Autodesk Inventor part; units mm, degrees
(part 7 of 7)
sketch "Esboço14" plane through (-80, -75, 4) normal (0, -1, 0) x (1, 0, 0)
  line L0 (170, 0) -> (160, 0) projected
  line L1 (160, 0) -> (160, -46)
  line L2 (160, -132) -> (160, 0) projected
  line L3 (160, 0) -> (206, 0) construction
  line L4 (160, -46) -> (0, -46)
  line L5 (0, 0) -> (0, -132) projected
  line L6 (160, -4) -> (160, 0) projected
  line L7 (160, 0) -> (160, -84)
  line L8 (160, 0) -> (244, 0) construction
  line L9 (160, -84) -> (0, -84)
  line L10 (160, -46) -> (160, -65)
  line L11 (160, -46) -> (179, -46) construction
  line L12 (160, -65) -> (125.67, -65)
  line L13 (125.67, -65) -> (103.67, -65)
  line L14 (103.67, -65) -> (69.34, -65)
  line L15 (69.34, -65) -> (34.34, -65)
  line L16 (69.34, -65) -> (104.34, -65) construction
  line L17 (34.34, -65) -> (0.01, -65)
  line L18 (124.67, -71.5) -> (104.67, -71.5)
  line L19 (104.67, -71.5) -> (104.67, -58.5)
  line L20 (104.67, -58.5) -> (124.67, -58.5)
  line L21 (124.67, -58.5) -> (124.67, -71.5)
  line L22 (124.67, -71.5) -> (104.67, -58.5) construction
  line L23 (104.67, -71.5) -> (124.67, -58.5) construction
  line L24 (62.24, -71.4) -> (41.44, -71.4)
  line L25 (41.44, -71.4) -> (41.44, -58.6)
  line L26 (41.44, -58.6) -> (62.24, -58.6)
  line L27 (62.24, -58.6) -> (62.24, -71.4)
  line L28 (62.24, -71.4) -> (41.44, -58.6) construction
  line L29 (41.44, -71.4) -> (62.24, -58.6) construction
  line L30 (160, -132) -> (160, -129)
  line L31 (160, -132) -> (163, -132) construction
  line L32 (160, -129) -> (0, -129)
  line L33 (160, -84) -> (160, -109.5)
  line L34 (160, -84) -> (185.5, -84) construction
  line L35 (160, -109.5) -> (150, -109.5)
  line L36 (150, -109.5) -> (85, -109.5)
  line L37 (85, -109.5) -> (65, -109.5)
  line L38 (65, -109.5) -> (53, -109.5)
  line L39 (117.5, -109.5) -> (117.5, -104.5)
  line L40 (140, -106.5) -> (95, -106.5)
  line L41 (95, -106.5) -> (95, -102.5)
  line L42 (95, -102.5) -> (140, -102.5)
  line L43 (140, -102.5) -> (140, -106.5)
  line L44 (140, -106.5) -> (95, -102.5) construction
  line L45 (95, -106.5) -> (140, -102.5) construction
  circle A0 centre (59, -109.5) radius 3.5
  point P0 (80, -4)
  point P1 (114.67, -65)
  point P2 (51.84, -65)
  dimension "d150" = 46
  dimension "d151" = 90
  dimension "d152" = 84
  dimension "d153" = 90
  dimension "d154" = 19
  dimension "d155" = 90
  dimension "d156" = 34.33
  dimension "d157" = 22
  dimension "d158" = 34.33
  dimension "d159" = 35
  dimension "d160" = 180
  dimension "d161" = 34.33
  dimension "d162" = 180
  dimension "d163" = 20
  dimension "d164" = 13
  dimension "d165" = 20.8
  dimension "d166" = 12.8
  dimension "d167" = 3
  dimension "d168" = 90
  dimension "d169" = 25.5
  dimension "d170" = 90
  dimension "d171" = 10
  dimension "d172" = 65
  dimension "d173" = 20
  dimension "d174" = 12
  dimension "d175" = 5
  dimension "d176" = 45
  dimension "d177" = 4
  dimension "d178" = 7
  constraints: 84 end point, 12 horizontal, 10 midpoint, 8 perpendicular, 6 equal length, 6 parallel, 6 point on line, 5 collinear, 1 centre point, 1 vertical
  measures "d150" distance of L0.end L1.end
  measures "d151" angle of L1 L3
  measures "d152" distance of L0.end L7.end
  measures "d153" angle of L7 L8
  measures "d154" distance of L1.end L10.end
  measures "d155" angle of L10 L11
  measures "d156" distance of L10.end L12.end
  measures "d157" distance of L12.end L13.end
  measures "d158" distance of L13.end L14.end
  measures "d159" distance of L14.end L15.end
  measures "d160" angle of L15 L16
  measures "d161" distance of L15.end L17.end
  measures "d162" angle of L17 L15
  measures "d163" distance of L19.end L20.end
  measures "d164" distance of L18.end L19.end
  measures "d165" distance of L25.end L26.end
  measures "d166" distance of L24.end L25.end
  measures "d167" distance of L2.start L30.end
  measures "d168" angle of L31 L30
  measures "d169" distance of L7.end L33.end
  measures "d170" angle of L33 L34
  measures "d171" distance of L33.end L35.end
  measures "d172" distance of L35.end L36.end
  measures "d173" distance of L36.end L37.end
  measures "d174" distance of L37.end L38.end
  measures "d175" distance of L39.start L39.end
  measures "d176" distance of L41.end L42.end
  measures "d177" distance of L40.end L41.end
  measures "d178" diameter of A0
extrude "Extrusão14" cut sketch "Esboço14" against normal blind 5 contours L21 L18 L19 L13 | L13 L19 L20 L21 | L27 L24 L25 L15 | L15 L25 L26 L27 | A0 L38 | L38 A0 | L40 L41 L42 L43
sketch "Esboço15" plane through (-80, -75, 4) normal (0, -1, 0) x (1, 0, 0)
  line L0 (170, 0) -> (160, 0)
  line L1 (160, 0) -> (160, -46)
  line L2 (160, -132) -> (160, 0)
  line L3 (160, 0) -> (206, 0) construction
  line L4 (160, -46) -> (0, -46)
  line L5 (0, 0) -> (0, -132)
  line L6 (160, -4) -> (160, 0)
  line L7 (160, 0) -> (160, -84)
  line L8 (160, 0) -> (244, 0) construction
  line L9 (160, -84) -> (0, -84)
  line L10 (160, -46) -> (160, -65)
  line L11 (160, -46) -> (179, -46) construction
  line L12 (160, -65) -> (125.67, -65)
  line L13 (125.67, -65) -> (103.67, -65)
  line L14 (103.67, -65) -> (69.34, -65)
  line L15 (69.34, -65) -> (34.34, -65)
  line L16 (69.34, -65) -> (104.34, -65) construction
  line L17 (34.34, -65) -> (0.01, -65)
  line L18 (124.67, -71.5) -> (104.67, -71.5)
  line L19 (104.67, -71.5) -> (104.67, -58.5)
  line L20 (104.67, -58.5) -> (124.67, -58.5)
  line L21 (124.67, -58.5) -> (124.67, -71.5)
  line L22 (124.67, -71.5) -> (104.67, -58.5) construction
  line L23 (104.67, -71.5) -> (124.67, -58.5) construction
  line L24 (62.24, -71.4) -> (41.44, -71.4)
  line L25 (41.44, -71.4) -> (41.44, -58.6)
  line L26 (41.44, -58.6) -> (62.24, -58.6)
  line L27 (62.24, -58.6) -> (62.24, -71.4)
  line L28 (62.24, -71.4) -> (41.44, -58.6) construction
  line L29 (41.44, -71.4) -> (62.24, -58.6) construction
  line L30 (160, -132) -> (160, -129)
  line L31 (160, -132) -> (163, -132) construction
  line L32 (160, -129) -> (0, -129)
  line L33 (160, -84) -> (160, -109.5)
  line L34 (160, -84) -> (185.5, -84) construction
  line L35 (160, -109.5) -> (150, -109.5)
  line L36 (150, -109.5) -> (85, -109.5)
  line L37 (85, -109.5) -> (65, -109.5)
  line L38 (65, -109.5) -> (53, -109.5)
  line L39 (117.5, -109.5) -> (117.5, -104.5)
  line L40 (140, -106.5) -> (95, -106.5)
  line L41 (95, -106.5) -> (95, -102.5)
  line L42 (95, -102.5) -> (140, -102.5)
  line L43 (140, -102.5) -> (140, -106.5)
  line L44 (140, -106.5) -> (95, -102.5) construction
  line L45 (95, -106.5) -> (140, -102.5) construction
  circle A0 centre (59, -109.5) radius 3.5
  line L46 (65.59, -65.5) -> (38.09, -65.5)
  line L47 (38.09, -65.5) -> (38.09, -64.5)
  line L48 (38.09, -64.5) -> (65.59, -64.5)
  line L49 (65.59, -64.5) -> (65.59, -65.5)
  line L50 (65.59, -65.5) -> (38.09, -64.5) construction
  line L51 (38.09, -65.5) -> (65.59, -64.5) construction
  circle A1 centre (65.59, -65) radius 1
  circle A2 centre (38.09, -65) radius 1
  line L52 (146.5, -110) -> (88.5, -110)
  line L53 (88.5, -110) -> (88.5, -109)
  line L54 (88.5, -109) -> (146.5, -109)
  line L55 (146.5, -109) -> (146.5, -110)
  line L56 (146.5, -110) -> (88.5, -109) construction
  line L57 (88.5, -110) -> (146.5, -109) construction
  circle A3 centre (146.5, -109.5) radius 1
  circle A4 centre (88.5, -109.5) radius 1
  point P0 (80, -4)
  point P1 (80, -4)
  point P2 (114.67, -65)
  point P3 (51.84, -65)
  dimension "d181" = 46
  dimension "d182" = 90
  dimension "d183" = 84
  dimension "d184" = 90
  dimension "d185" = 19
  dimension "d186" = 90
  dimension "d187" = 34.33
  dimension "d188" = 22
  dimension "d189" = 34.33
  dimension "d190" = 35
  dimension "d191" = 180
  dimension "d192" = 34.33
  dimension "d193" = 180
  dimension "d194" = 20
  dimension "d195" = 13
  dimension "d196" = 20.8
  dimension "d197" = 12.8
  dimension "d198" = 3
  dimension "d199" = 90
  dimension "d200" = 25.5
  dimension "d201" = 90
  dimension "d202" = 10
  dimension "d203" = 65
  dimension "d204" = 20
  dimension "d205" = 12
  dimension "d206" = 5
  dimension "d207" = 45
  dimension "d208" = 4
  dimension "d209" = 7
  dimension "d210" = 27.5
  dimension "d211" = 1
  dimension "d212" = 2
  dimension "d213" = 2
  dimension "d214" = 58
  dimension "d215" = 1
  dimension "d216" = 2
  dimension "d217" = 2
  constraints: 116 end point, 18 midpoint, 14 horizontal, 10 parallel, 10 perpendicular, 6 equal length, 6 point on line, 5 centre point, 5 collinear, 1 vertical
  measures "d181" distance of L0.end L1.end
  measures "d182" angle of L1 L3
  measures "d183" distance of L0.end L7.end
  measures "d184" angle of L7 L8
  measures "d185" distance of L1.end L10.end
  measures "d186" angle of L10 L11
  measures "d187" distance of L10.end L12.end
  measures "d188" distance of L12.end L13.end
  measures "d189" distance of L13.end L14.end
  measures "d190" distance of L14.end L15.end
  measures "d191" angle of L15 L16
  measures "d192" distance of L15.end L17.end
  measures "d193" angle of L17 L15
  measures "d194" distance of L19.end L20.end
  measures "d195" distance of L18.end L19.end
  measures "d196" distance of L25.end L26.end
  measures "d197" distance of L24.end L25.end
  measures "d198" distance of L2.start L30.end
  measures "d199" angle of L31 L30
  measures "d200" distance of L7.end L33.end
  measures "d201" angle of L33 L34
  measures "d202" distance of L33.end L35.end
  measures "d203" distance of L35.end L36.end
  measures "d204" distance of L36.end L37.end
  measures "d205" distance of L37.end L38.end
  measures "d206" distance of L39.start L39.end
  measures "d207" distance of L41.end L42.end
  measures "d208" distance of L40.end L41.end
  measures "d209" diameter of A0
  measures "d210" distance of L47.end L48.end
  measures "d211" distance of L46.end L47.end
  measures "d212" diameter of A1
  measures "d213" diameter of A2
  measures "d214" distance of L53.end L54.end
  measures "d215" distance of L52.end L53.end
  measures "d216" diameter of A3
  measures "d217" diameter of A4
extrude "Extrusão15" cut sketch "Esboço15" against normal blind 5 contours A1 L46 L49 L15 | L15 L49 L48 A1 | L49 L46 A1 L15 | L15 A1 L48 L49 | A2 L15 L47 L48 | L48 L47 L15 A2 | A2 L15 L47 L46 | L46 L47 L15 A2 | A4 L52 L53 L36 | L36 L53 L54 A4 | A3 L54 L55 L36 | L36 L55 L52 A3 | L53 L52 A4 L36 | L36 A4 L54 L53 | L55 L54 A3 L36 | L36 A3 L52 L55
sketch "Esboço17" plane through (-64.7396, -70, 0) normal (0, 1, 0) x (1, 0, 0)
  line L0 (36.7396, 111.5) -> (50.7396, 111.5)
  line L1 (50.7396, 111.5) -> (50.7396, 99.5)
  line L2 (50.7396, 99.5) -> (36.7396, 99.5)
  line L3 (36.7396, 99.5) -> (36.7396, 111.5)
  circle A0 centre (43.7396, 105.5) radius 3.5 projected
  line L4 (36.7396, 111.5) -> (50.7396, 99.5) construction
  line L5 (50.7396, 111.5) -> (36.7396, 99.5) construction
  point P0 (64.7396, 0)
  dimension "d222" = 14
  dimension "d223" = 12
  constraints: 12 end point, 2 midpoint, 2 parallel, 1 horizontal, 1 perpendicular
  measures "d222" distance of L1.end L2.end
  measures "d223" distance of L0.end L1.end
extrude "Extrusão17" cut sketch "Esboço17" against normal blind 3
sketch "Esboço18" plane through (-80, 75, 4) normal (0, 1, 0) x (1, 0, 0)
  arc A0 (72.5485, 53.3799) -> (79.9881, 42.7636) centre (85.5481, 54.5748) ccw
  line L0 (79.9881, 55.0366) -> (79.9881, 58.2133)
  arc A1 (79.2401, 48.9381) -> (73.734, 53.3799) centre (74.6193, 48.8437) ccw
  arc A2 (73.734, 53.3799) -> (79.2401, 48.9381) centre (78.3806, 53.5063) ccw
  arc A3 (79.9881, 42.7636) -> (87.4277, 53.3799) centre (74.4281, 54.5748) ccw
  arc A4 (86.2422, 53.3799) -> (80.7361, 48.9381) centre (85.3569, 48.8437) ccw
  arc A5 (80.7361, 48.9381) -> (86.2422, 53.3799) centre (81.5956, 53.5063) ccw
  arc A6 (87.4277, 53.3799) -> (72.5485, 53.3799) centre (79.9881, 54.6819) ccw
  arc A7 (79.9881, 58.2133) -> (79.9932, 51.0786) centre (82.9707, 54.6481) ccw
  arc A8 (79.9932, 51.0786) -> (79.9881, 58.2133) centre (77.0522, 54.6438) ccw
  circle A9 centre (53.34, 108) radius 6.75 projected
  line L1 (53.34, 101.25) -> (53.34, 0)
  line L2 (44.1532, 0) -> (57.5876, 0) projected
  line L3 (0, 50.625) -> (159.975, 50.625)
  arc A10 (80.0139, 41.108) -> (88.645, 53.4246) centre (73.5634, 54.8108) ccw
  line L4 (80.0236, 66.3313) -> (80.0236, 64.8313)
  line L5 (80.0139, 41.108) -> (80.0139, 43.361)
  arc A11 (71.3827, 53.4246) -> (80.0139, 41.108) centre (86.4643, 54.8108) ccw
  arc A12 (88.645, 53.4246) -> (71.3827, 53.4246) centre (80.0139, 54.9348) ccw
  point P0 (80, 4)
  point P1 (79.9618, 50.6395)
  point P2 (80.0144, 50.6395)
  point P3 (87.4372, 53.423)
  point P4 (79.9881, 62.2346)
  point P5 (53.34, 50.625)
  point P6 (79.9875, 50.625)
  point P7 (0, 0)
  point P8 (0, 0)
  point P9 (80.0048, 63.284)
  point P10 (0, 0)
  point P11 (0, 0)
  point P12 (0, 0)
  point P13 (0, 0)
  point P14 (80.0005, 64.548)
  point P15 (79.9985, 63.697)
  dimension "d226" = 19.471
  dimension "d227" = 23.44
  dimension "d228" = 1.5
  constraints: 27 point on circle, 12 centre point, 10 end point, 8 symmetric about line, 2 midpoint, 1 point on line, 1 vertical, 1 vertical alignment, 5 other
  measures "d226" distance of A0.end point (79.988, 62.235)
  measures "d227" distance of L5.start point (80.001, 64.548)
  measures "d228" distance of L4.start L4.end
extrude "Extrusão18" cut sketch "Esboço18" against normal blind 2 contours A6 A3 L3 A5 A4 A1 A2 A0 | A0 L3 A11 A12 A10 A3 A6 | L3 A2 A1 A4 A5 A3 A0 | A0 A3 L5 A11 L3 | L3 A1 A2 | A2 A1 L3 | L3 A10 L5 A3 | L3 A4 A5 | A5 A4 L3 | A8 A7
